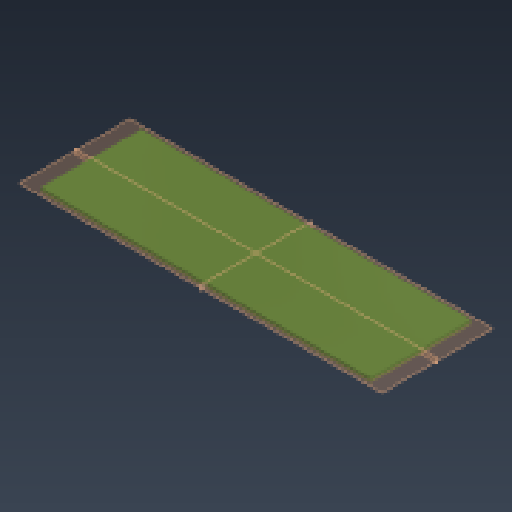
# Autodesk Inventor part: Фанерка_аккумуляторов
Saved by Autodesk Inventor 2023.2 (Build 272271030, 271C)
## iProperties
Created: 2025-12-29
Part Number: Фанерка_аккумуляторов
Material: Типовые
Document SubType Name: Modeling
Designer: Олег Коноваленко
Density: 1 g/cm^3
Appearance: Темно-оливковый
Author: Олег Коноваленко
Autodesk Inventor part; units mm, degrees
sketch "Эскиз1" plane through (0, 0, 0) normal (0, 1, 0) x (-1, 0, 0)
  line L0 (147, 45) -> (-147, 45)
  line L1 (-147, 45) -> (-147, -45)
  line L2 (-147, -45) -> (147, -45)
  line L3 (147, -45) -> (147, 45)
  line L4 (147, 45) -> (-147, -45) construction
  line L5 (-147, 45) -> (147, -45) construction
  point P0 (0, 0)
  dimension "d3" = 294
  dimension "d4" = 90
  constraints: 12 end point, 2 midpoint, 2 parallel, 1 horizontal, 1 perpendicular
  measures "d3" distance of L1.end L2.end
  measures "d4" distance of L0.end L1.end
extrude "Выдавливание1" add sketch "Эскиз1" along normal mid plane 4
sketch "Эскиз2" plane through (0, 2, 0) normal (0, 1, 0) x (1, 0, 0)
  line L0 (-127, -35) -> (-127, -30) projected
  line L1 (-127, -30) -> (-142, -30) projected
  line L2 (-142, -30) -> (-142, -35) projected
  line L3 (-142, -35) -> (-127, -35) projected
  line L4 (-102, -35) -> (-102, -30) projected
  line L5 (-102, -30) -> (-117, -30) projected
  line L6 (-117, -30) -> (-117, -35) projected
  line L7 (-117, -35) -> (-102, -35) projected
  line L8 (102, -35) -> (102, -30) projected
  line L9 (117, -35) -> (102, -35) projected
  line L10 (117, -30) -> (117, -35) projected
  line L11 (102, -30) -> (117, -30) projected
  line L12 (127, -35) -> (127, -30) projected
  line L13 (142, -35) -> (127, -35) projected
  line L14 (142, -30) -> (142, -35) projected
  line L15 (127, -30) -> (142, -30) projected
  circle A0 centre (122, -32.5) radius 2 projected
  circle A1 centre (-122, -32.5) radius 2 projected
  point P0 (0, 0)
extrude "Выдавливание2" cut sketch "Эскиз2" against normal up to next
sketch "Эскиз3" plane through (0, 2, 0) normal (0, 1, 0) x (1, 0, 0)
  line L0 (80, 0) -> (-80, 0) construction
  line L1 (80, 15) -> (-80, 15)
  line L2 (-80, -15) -> (80, -15)
  arc A0 (80, -15) -> (80, 15) centre (80, 0) ccw
  arc A1 (-80, 15) -> (-80, -15) centre (-80, 0) ccw
  line L3 (55, -15) -> (30, -15)
  line L4 (30, -15) -> (30, 15)
  line L5 (30, 15) -> (55, 15)
  line L6 (55, 15) -> (55, -15)
  line L7 (-29, -15) -> (-54, -15)
  line L8 (-54, -15) -> (-54, 15)
  line L9 (-54, 15) -> (-29, 15)
  line L10 (-29, 15) -> (-29, -15)
  line L11 (-44, -11) -> (-44, -1) projected
  line L12 (40, -11) -> (40, -1) projected
  point P0 (0, 0)
  point P1 (-29, 15)
  dimension "d7" = 160
  dimension "d8" = 15
  dimension "d11" = 25
  dimension "d12" = 25
  dimension "d13" = 10
  dimension "d14" = 10
  constraints: 24 end point, 5 parallel, 4 point on circle, 4 point on line, 4 tangent, 3 horizontal, 2 centre point, 2 perpendicular, 1 midpoint
  measures "d7" distance of L0.start L0.end
  measures "d8" distance between parallel lines of L2 L0
  measures "d11" distance between parallel lines of L4 L6
  measures "d12" distance between parallel lines of L8 L10
  measures "d13" distance between parallel lines of L4 L12
  measures "d14" distance between parallel lines of L8 L11
extrude "Выдавливание3" cut sketch "Эскиз3" against normal up to next contours A0 L2 L6 L1 | L4 L2 L10 L1 | L8 L2 A1 L1
sketch "Эскиз4" plane through (0, 2, 0) normal (0, 1, 0) x (1, 0, 0)
  line L0 (40, -21) -> (44, -21) projected
  line L1 (44, -21) -> (44, -31) projected
  line L2 (40, -31) -> (40, -21) projected
  line L3 (40, -31) -> (44, -31) projected
  line L4 (44, -11) -> (40, -11) projected
  line L5 (44, -1) -> (44, -11) projected
  line L6 (40, -1) -> (44, -1) projected
  line L7 (40, -11) -> (40, -1) projected
  line L8 (-44, -21) -> (-40, -21) projected
  line L9 (-44, -31) -> (-44, -21) projected
  line L10 (-44, -31) -> (-40, -31) projected
  line L11 (-40, -21) -> (-40, -31) projected
  line L12 (-40, -11) -> (-44, -11) projected
  line L13 (-40, -1) -> (-40, -11) projected
  line L14 (-44, -1) -> (-40, -1) projected
  line L15 (-44, -11) -> (-44, -1) projected
  circle A0 centre (42, -16) radius 1.5
  circle A1 centre (-42, -16) radius 1.5
  line L16 (-42, 24.8) -> (-42, -50.8) construction
  line L17 (42, 24.8) -> (42, -50.8) construction
  point P0 (0, 0)
  dimension "d15" = 3
  dimension "d16" = 5
  dimension "d17" = 5
  constraints: 4 end point, 2 centre point, 2 point on line, 2 vertical, 1 equal radius, 4 other
  measures "d15" diameter of A1
  measures "d16" distance from line of L8 A1.centre
  measures "d17" distance from line of L0 A0.centre
extrude "Выдавливание4" cut sketch "Эскиз4" against normal up to next
fillet "Сопряжение1" radius 3 10 edges at (55, 0, 15) (55, 0, -15) (-29, 0, 15) (-29, 0, -15) (30, 0, -15) (30, 0, 15) (-54, 0, 15) (-54, 0, -15) (147, 0, -45) (-147, 0, -45)
sketch "Эскиз5" plane through (0, 2, 0) normal (0, 1, 0) x (1, 0, 0)
  spline S0 degree 3 poles (0.1, 32.25) (-0.0887, 32.25) (-0.2898, 32.2122) (-0.6592, 32.059) (-0.8277, 31.9436) (-1.0936, 31.6777) (-1.209, 31.5092) (-1.3622, 31.1398) (-1.4, 30.9387) (-1.4, 30.5613) (-1.3622, 30.3602) (-1.209, 29.9908) (-1.0936, 29.8223) (-0.8277, 29.5564) (-0.6592, 29.441) (-0.2898, 29.2878) (-0.0887, 29.25) (0.2887, 29.25) (0.4898, 29.2878) (0.8592, 29.441) (1.0277, 29.5564) (1.2936, 29.8223) (1.409, 29.9908) (1.5622, 30.3602) (1.6, 30.5613) (1.6, 30.9387) (1.5622, 31.1398) (1.409, 31.5092) (1.2936, 31.6777) (1.0277, 31.9436) (0.8592, 32.059) (0.4898, 32.2122) (0.2887, 32.25) (0.1, 32.25) knots -0.905867 -0.905867 -0.905867 -0.905867 -0.84925 -0.84925 -0.792632 -0.792632 -0.736016 -0.736016 -0.6794 -0.6794 -0.622784 -0.622784 -0.566168 -0.566168 -0.509551 -0.509551 -0.452934 -0.452934 -0.396316 -0.396316 -0.339699 -0.339699 -0.283083 -0.283083 -0.226467 -0.226467 -0.169851 -0.169851 -0.113235 -0.113235 -0.056617 -0.056617 0 0 0 0 projected
  spline S1 degree 3 poles (0.1, -29.25) (-0.0887, -29.25) (-0.2898, -29.2878) (-0.6592, -29.441) (-0.8277, -29.5564) (-1.0936, -29.8223) (-1.209, -29.9908) (-1.3622, -30.3602) (-1.4, -30.5613) (-1.4, -30.9387) (-1.3622, -31.1398) (-1.209, -31.5092) (-1.0936, -31.6777) (-0.8277, -31.9436) (-0.6592, -32.059) (-0.2898, -32.2122) (-0.0887, -32.25) (0.2887, -32.25) (0.4898, -32.2122) (0.8592, -32.059) (1.0277, -31.9436) (1.2936, -31.6777) (1.409, -31.5092) (1.5622, -31.1398) (1.6, -30.9387) (1.6, -30.5613) (1.5622, -30.3602) (1.409, -29.9908) (1.2936, -29.8223) (1.0277, -29.5564) (0.8592, -29.441) (0.4898, -29.2878) (0.2887, -29.25) (0.1, -29.25) knots -0.905867 -0.905867 -0.905867 -0.905867 -0.84925 -0.84925 -0.792632 -0.792632 -0.736016 -0.736016 -0.6794 -0.6794 -0.622784 -0.622784 -0.566168 -0.566168 -0.509551 -0.509551 -0.452934 -0.452934 -0.396316 -0.396316 -0.339699 -0.339699 -0.283083 -0.283083 -0.226467 -0.226467 -0.169851 -0.169851 -0.113235 -0.113235 -0.056617 -0.056617 0 0 0 0 projected
  point P0 (0, 0)
  point P1 (0.1, 32.25)
  point P2 (0.1, -29.25)
extrude "Выдавливание5" cut sketch "Эскиз5" against normal up to next
